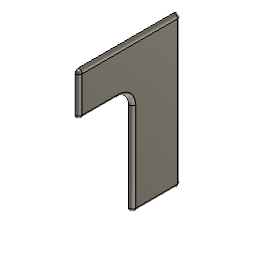
Fusion360ModelofIRClinicalThermo (Autodesk Fusion 360 archive; units mm, degrees)
design "kapak_yeni"
part number: 2026-05-16-18-50-38-816
Autodesk Fusion 360 part; units mm, degrees
sketch "Çizim1" plane through (0, 0, 0) normal (1, 0, 0) x (0, 1, 0)
  line L0 (0, 90) -> (0, 0)
  line L1 (-45, 123) -> (35, 123)
  line L2 (35, -3) -> (0, -3)
  line L3 (35, 120) -> (-45, 120)
  arc A0 (38, 120) -> (35, 123) centre (35, 120) ccw
  line L4 (-45, 87) -> (-15, 87)
  line L5 (38, 120) -> (38, 0)
  line L6 (-3, 0) -> (-3, 75)
  line L7 (-45, 120) -> (-45, 90)
  line L8 (-48, 90) -> (-48, 120)
  arc A1 (-3, 0) -> (0, -3) centre (0, 0) ccw
  arc A2 (35, -3) -> (38, 0) centre (35, 0) ccw
  arc A3 (-45, 123) -> (-48, 120) centre (-45, 120) ccw
  arc A4 (-3, 75) -> (-15, 87) centre (-15, 75) ccw
  arc A5 (-48, 90) -> (-45, 87) centre (-45, 90) ccw
  line L9 (35, 0) -> (35, 120)
  line L10 (0, 0) -> (35, 0)
  line L11 (-45, 90) -> (0, 90)
  point P0 (38, 123)
  point P1 (-48, 87)
  point P2 (-48, 123)
  point P3 (-3, -3)
  point P4 (38, -3)
  dimension "d1" = 35
  dimension "d2" = 120
  dimension "d3" = 3
  dimension "d4" = 36
  dimension "d5" = 86
  dimension "d6" = 126
  dimension "d7" = 41
  dimension "d8" = 3
  dimension "d9" = 3
  dimension "d10" = 3
  dimension "d11" = 3
  dimension "d12" = 3
  dimension "d13" = 12
  constraint coincident L0.end A1.centre
  constraint horizontal L10
  constraint perpendicular L9 L10
  constraint perpendicular L3 L9
  constraint perpendicular L3 L7
  constraint perpendicular L7 L11
  constraint perpendicular L0 L10
  constraint perpendicular L0 L4
  constraint perpendicular L1 L8
  constraint perpendicular L3 L5
  constraint perpendicular L2 L8
  constraint perpendicular L4 L6
  constraint coincident P2 L8
  constraint coincident P2 L1
  constraint tangent L8 A3
  constraint tangent L1 A3
  constraint coincident P1 L8
  constraint tangent L8 A5
  constraint coincident L4.start A5.end
  constraint coincident P0 L1
  constraint coincident P0 L5
  constraint tangent L1 A0
  constraint tangent A0 L5
  constraint coincident P4 L5
  constraint coincident P4 L2
  constraint tangent L5 A2
  constraint tangent L2 A2
  constraint coincident P3 L2
  constraint coincident P3 L6
  constraint tangent L2 A1
  constraint tangent L6 A1
  constraint tangent L6 A4
  constraint tangent L4 A4
  measures "d1" distance of L0.end A2.centre
  measures "d2" distance of L3.start A2.centre
  measures "d3" distance of L7.end L4.start
  measures "d4" distance of P1 P2
  measures "d5" distance of P0 P2
  measures "d6" distance of P0 P4
  measures "d7" distance of P3 P4
  measures "d8" radius of A3
  measures "d9" radius of A5
  measures "d10" radius of A0
  measures "d11" radius of A2
  measures "d12" radius of A1
  measures "d13" radius of A4
extrude "Ekstrüzyon1" add sketch "Çizim1" along normal blind 3 contours L0 L3 L7 L9 L10 L11 | L1 L2 A0 L4 L5 L6 L8 A1 A2 A3 A4 A5
fillet "Fillet1" radius 3 12 edges at (3, -48, 105) (3, -47.1213, 87.8787) (3, -30, 87) (3, -6.5147, 83.4853) (3, -3, 37.5) (3, -2.1213, -2.1213) (3, 17.5, -3) (3, 37.1213, -2.1213) (3, 38, 60) (3, 37.1213, 122.1213) (3, -5, 123) (3, -47.1213, 122.1213)
